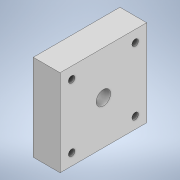
# Autodesk Inventor part: nut_blocker
Saved by Autodesk Inventor 2020 (Build 240168000, 168)
## iProperties
Created: 2019-12-27
Part Number: nut_blocker
Material: Générique
Document SubType Name: Modeling
Designer: damien
Density: 1 g/cm^3
Appearance: Par défaut
Author: damien
Autodesk Inventor part; units mm, degrees
ref_plane "YZ Plane" through (0, 0, 0) normal (1, 0, 0) x (0, 1, 0)
ref_plane "XZ Plane" through (0, 0, 0) normal (0, 1, 0) x (-1, 0, 0)
ref_plane "XY Plane" through (0, 0, 0) normal (0, 0, 1) x (1, 0, 0)
sketch "Esquisse1" plane through (0, 0, 0) normal (1, 0, 0) x (0, 1, 0)
  line L0 (-30, -30) -> (30, -30)
  line L1 (30, -30) -> (30, 30)
  line L2 (30, 30) -> (-30, 30)
  line L3 (-30, 30) -> (-30, -30)
  line L4 (-30, -30) -> (30, 30) construction
  line L5 (30, -30) -> (-30, 30) construction
  circle A0 centre (22, 22) radius 2.25
  circle A1 centre (-22, 22) radius 2.25
  circle A2 centre (22, -22) radius 2.25
  circle A3 centre (-22, -22) radius 2.25
  point P0 (0, 0)
  dimension "d0" = 60
  dimension "d1" = 8
  dimension "d2" = 4.5
  constraints: 12 end point, 4 centre point, 4 point on line, 3 equal radius, 2 horizontal alignment, 2 midpoint, 2 parallel, 2 perpendicular, 2 vertical alignment, 1 horizontal
  measures "d0" distance of L0.end L1.end
  measures "d1" distance from line of L1 A0.centre
  measures "d2" diameter of A0
extrude "Extrusion1" add sketch "Esquisse1" along normal blind 18.55
sketch "Esquisse2" plane through (18.55, 0, 0) normal (1, 0, 0) x (0, 0, -1)
  circle A0 centre (0, 0) radius 5
  dimension "d5" = 10
  constraints: 1 centre point, 1 coincident
  measures "d5" diameter of A0
extrude "Extrusion2" cut sketch "Esquisse2" against normal blind 18.55
